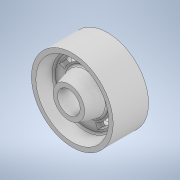
# Autodesk Inventor part: roller
Saved by Autodesk Inventor 2021 (Build 250183000, 183)
## iProperties
Created: 2022-04-24
Part Number: roller
Material: Generic
Document SubType Name: Modeling
Designer: hp
Density: 1 g/cm^3
Appearance: Default
Author: hp
Autodesk Inventor part; units mm, degrees
ref_plane "YZ Plane" through (0, 0, 0) normal (1, 0, 0) x (0, 1, 0)
ref_plane "XZ Plane" through (0, 0, 0) normal (0, 1, 0) x (-1, 0, 0)
sketch "Sketch1" plane through (0, 0, 0) normal (1, 0, 0) x (0, 1, 0)
  line L0 (0, 0) -> (4.5, 0)
  line L1 (4.5, 0) -> (4.5, 43)
  line L2 (4.5, 43) -> (0, 43)
  line L3 (0, 43) -> (0, 0)
  line L4 (4.5, 43) -> (8.9259, 26.4824)
  line L5 (4.5, 21.5) -> (10.3528, 21.5)
  line L6 (13, 25) -> (10.8577, 25)
  line L7 (25.5, 39.5) -> (30, 39.5)
  line L8 (30, 39.5) -> (30, 3.5)
  line L9 (30, 3.5) -> (25.5, 3.5)
  line L10 (25.5, 3.5) -> (25.5, 39.5)
  line L11 (25.5, 39.5) -> (22.0119, 26.4824)
  line L12 (10.8577, 18) -> (20.0801, 18)
  line L13 (4.5, 0) -> (8.9259, 16.5176)
  line L14 (25.5, 3.5) -> (22.0119, 16.5176)
  line L15 (3, 25) -> (20.0801, 25)
  arc A0 (8.9259, 26.4824) -> (10.8577, 25) centre (10.8577, 27) ccw
  arc A1 (20.0801, 25) -> (22.0119, 26.4824) centre (20.0801, 27) ccw
  arc A2 (22.0119, 16.5176) -> (20.0801, 18) centre (20.0801, 16) ccw
  arc A3 (10.8577, 18) -> (8.9259, 16.5176) centre (10.8577, 16) ccw
  line L16 (-11.5, 16.5176) -> (-11.5, 3.5)
  point P0 (9.6974, 23.6032)
  point P1 (21.6069, 24.9709)
  point P2 (3, 18)
  point P3 (23.25, 18)
  point P4 (9.6974, 19.3968)
  point P5 (21.6069, 18.0291)
  point P6 (23.25, 25)
  dimension "d0" = 43
  dimension "d1" = 4.5
  dimension "d2" = 15
  dimension "d3" = 21.5
  dimension "d4" = 3.5
  dimension "d5" = 4.5
  dimension "d6" = 36
  dimension "d7" = 18
  dimension "d8" = 15
  dimension "d9" = 3.5
  dimension "d10" = 30
  dimension "d11" = 2
  dimension "d12" = 32
  constraints: 34 end point, 8 point on circle, 8 tangent, 7 point on line, 4 centre point, 4 horizontal, 4 parallel, 4 symmetric about line, 3 equal radius, 2 perpendicular, 1 midpoint, 1 vertical
  measures "d0" distance of L2.end L0.start
  measures "d1" distance of L0.start L0.end
  measures "d2" angle of L1 L4
  measures "d3" distance from line of L0.start L5
  measures "d4" distance between parallel lines of L6 L5
  measures "d5" distance between parallel lines of L8 L10
  measures "d6" distance of L7.end L8.end
  measures "d7" distance between parallel lines of L7 L5
  measures "d8" angle of L10 L11
  measures "d9" distance between parallel lines of L5 L12
  measures "d10" distance between parallel lines of L3 L8
  measures "d11" radius of A0
  measures "d12" diameter of L1 L16
revolve "Revolution1" add sketch "Sketch1" angle 360 about axis through (0, -11.5, 16.5176) along (0, 0, -1)
ref_plane "Work Plane1" through (0, -11.5, 75) normal (0, 0, 1) x (1, 0, 0)
sketch "Sketch2" plane through (0, -11.5, 75) normal (0, 0, 1) x (1, 0, 0)
  line L0 (9.2559, 22.3457) -> (12.1824, 29.4109)
  line L1 (22.3457, 9.2559) -> (27.1721, 11.2551)
  line L2 (0, 0) -> (0, 29.4109)
  line L3 (0, 0) -> (29.4109, 0)
  arc A0 (27.3903, 11.3454) -> (11.3454, 27.3903) centre (0, 0) ccw
  line L4 (22.3457, 9.2559) -> (27.1721, 11.2551)
  line L5 (22.3457, 9.2559) -> (27.3903, 11.3454)
  line L6 (22.3457, 9.2559) -> (27.3903, 11.3454)
  arc A1 (22.3457, 9.2559) -> (9.2559, 22.3457) centre (0, 0) ccw
  arc A2 (0, 24.1868) -> (24.1868, 0) centre (0, 0) ccw
  line L7 (11.3454, 27.3903) -> (9.2559, 22.3457)
  line L8 (27.3903, 11.3454) -> (22.3457, 9.2559)
  arc A3 (22.3457, 9.2559) -> (9.2559, 22.3457) centre (0, 0) ccw
  arc A4 (27.3903, 11.3454) -> (11.3454, 27.3903) centre (0, 0) ccw
  line L9 (9.2559, -22.3457) -> (12.1824, -29.4109)
  line L10 (22.3457, -9.2559) -> (27.1721, -11.2551)
  arc A5 (11.3454, -27.3903) -> (27.3903, -11.3454) centre (0, 0) ccw
  line L11 (22.3457, -9.2559) -> (27.1721, -11.2551)
  line L12 (22.3457, -9.2559) -> (27.3903, -11.3454)
  line L13 (22.3457, -9.2559) -> (27.3903, -11.3454)
  arc A6 (9.2559, -22.3457) -> (22.3457, -9.2559) centre (0, 0) ccw
  line L14 (11.3454, -27.3903) -> (9.2559, -22.3457)
  line L15 (27.3903, -11.3454) -> (22.3457, -9.2559)
  arc A7 (9.2559, -22.3457) -> (22.3457, -9.2559) centre (0, 0) ccw
  arc A8 (11.3454, -27.3903) -> (27.3903, -11.3454) centre (0, 0) ccw
  line L16 (0, 0) -> (0, -24.1868)
  line L17 (-9.2559, 22.3457) -> (-12.1824, 29.4109)
  line L18 (-22.3457, 9.2559) -> (-27.1721, 11.2551)
  arc A9 (-11.3454, 27.3903) -> (-27.3903, 11.3454) centre (0, 0) ccw
  line L19 (-22.3457, 9.2559) -> (-27.1721, 11.2551)
  line L20 (-22.3457, 9.2559) -> (-27.3903, 11.3454)
  line L21 (-22.3457, 9.2559) -> (-27.3903, 11.3454)
  arc A10 (-9.2559, 22.3457) -> (-22.3457, 9.2559) centre (0, 0) ccw
  line L22 (-11.3454, 27.3903) -> (-9.2559, 22.3457)
  line L23 (-27.3903, 11.3454) -> (-22.3457, 9.2559)
  arc A11 (-9.2559, 22.3457) -> (-22.3457, 9.2559) centre (0, 0) ccw
  arc A12 (-11.3454, 27.3903) -> (-27.3903, 11.3454) centre (0, 0) ccw
  line L24 (-22.3457, -9.2559) -> (-27.1721, -11.2551)
  line L25 (-22.3457, -9.2559) -> (-27.1721, -11.2551)
  line L26 (-22.3457, -9.2559) -> (-27.3903, -11.3454)
  line L27 (-22.3457, -9.2559) -> (-27.3903, -11.3454)
  line L28 (-27.3903, -11.3454) -> (-22.3457, -9.2559)
  arc A13 (-22.3457, -9.2559) -> (-9.2559, -22.3457) centre (0, 0) ccw
  arc A14 (-22.3457, -9.2559) -> (-9.2559, -22.3457) centre (0, 0) ccw
  arc A15 (-27.3903, -11.3454) -> (-11.3454, -27.3903) centre (0, 0) ccw
  line L29 (-11.3454, -27.3903) -> (-9.2559, -22.3457)
  line L30 (-9.2559, -22.3457) -> (-12.1824, -29.4109)
  arc A16 (-27.3903, -11.3454) -> (-11.3454, -27.3903) centre (0, 0) ccw
  point P0 (0, 11.5)
  point P1 (-29.4109, 0)
  point P2 (-24.1868, 0)
  point P3 (-9.2559, 22.3457)
  point P4 (9.2559, -22.3457)
  point P5 (27.1721, -11.2551)
  point P6 (22.3457, -9.2559)
  point P7 (-22.3457, -9.2559)
  point P8 (-27.1721, -11.2551)
  dimension "d15" = 29.4109
  dimension "d16" = 22.5
  dimension "d17" = 22.5
  constraints: 62 end point, 35 point on circle, 20 symmetric about line, 17 centre point, 6 point on line, 5 coincident, 4 concentric, 2 collinear, 2 vertical, 1 perpendicular, 12 other
  measures "d15" vertical distance of L2.start L0.end
  measures "d16" angle of L0 L2
  measures "d17" angle of L1 L3
extrude "Extrusion1" cut sketch "Sketch2" against normal through all contours L0 A0 L5 L1 A1 | A2 L18 L20 A9 L17 | L10 L12 A5 L9 A2 | L29 A15 L26 L24 A2
equation "\"d3\" = 0.5 * d0"
equation "\"d7\" = 0.5 * d6"
body "Solid1"
